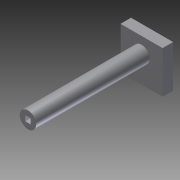
# Autodesk Inventor part: linac arm2
Saved by Autodesk Inventor 2011 (Build 150239000, 239)
## iProperties
Created: 2011-10-08
Part Number: linac arm2
Document SubType Name: Modeling
Designer: Matthew
Density: 1 g/cm^3
Author: Matthew
Autodesk Inventor part; units mm, degrees
ref_plane "YZ Plane" through (0, 0, 0) normal (1, 0, 0) x (0, 1, 0)
ref_plane "XZ Plane" through (0, 0, 0) normal (0, 1, 0) x (-1, 0, 0)
ref_plane "XY Plane" through (0, 0, 0) normal (0, 0, 1) x (1, 0, 0)
sketch "Sketch1" plane through (0, 0, 0) normal (0, 0, 1) x (1, 0, 0)
  circle A0 centre (0, 0) radius 9.906
  dimension "d0" = 19.812
  constraints: 1 centre point, 1 coincident
  measures "d0" diameter of A0
extrude "Extrusion1" add sketch "Sketch1" along normal blind 149.86
sketch "Sketch2" plane through (0, 0, 149.86) normal (0, 0, 1) x (1, 0, 0)
  circle A0 centre (0, 0) radius 9.906 projected
  circle A1 centre (0, 0) radius 3.175
  line L0 (-3.175, 0) -> (0, 0)
  line L1 (0, 0) -> (0, 3.175)
  line L2 (0, 3.175) -> (-3.175, 3.175)
  line L3 (-3.175, 3.175) -> (-3.175, 0)
  line L4 (-3.175, 3.175) -> (3.175, 3.175)
  line L5 (3.175, 3.175) -> (3.175, -3.175)
  line L6 (3.175, -3.175) -> (-3.175, -3.175)
  line L7 (-3.175, -3.175) -> (-3.175, 3.175)
  dimension "d3" = 6.35
  constraints: 16 end point, 4 parallel, 2 horizontal, 2 perpendicular, 2 point on circle, 1 centre point, 1 coincident
  measures "d3" diameter of A1
extrude "Extrusion2" cut sketch "Sketch2" against normal blind 12.7 contours A1 L0 L1 | L5 L6 A1 | A1 L4 L5 | L1 L0 A1 | A1 L3 L2 | L6 L7 A1
sketch "Sketch3" plane through (0, 0, 0) normal (0, 0, -1) x (-1, 0, 0)
  circle A0 centre (0, 0) radius 9.906 projected
  line L0 (0, 0) -> (-25.4, 0)
  line L1 (-25.4, 0) -> (-25.4, 25.4)
  line L2 (-25.4, 25.4) -> (0, 25.4)
  line L3 (0, 25.4) -> (0, 0)
  line L4 (-25.4, 25.4) -> (25.4, 25.4)
  line L5 (25.4, 25.4) -> (25.4, -25.4)
  line L6 (25.4, -25.4) -> (-25.4, -25.4)
  line L7 (-25.4, -25.4) -> (-25.4, 25.4)
  dimension "d6" = 25.4
  dimension "d7" = 25.4
  dimension "d8" = 50.8
  dimension "d9" = 50.8
  constraints: 16 end point, 4 parallel, 2 horizontal, 2 perpendicular
  measures "d6" distance of L1.end L2.end
  measures "d7" distance of L0.end L1.end
  measures "d8" distance of L5.end L6.end
  measures "d9" distance of L4.end L5.end
extrude "Extrusion3" add sketch "Sketch3" against normal blind 12.7 contours A0 L3 L4 L5 L6 L7 L0 | A0 L0 L1 L2 L3
sketch "Sketch4" plane through (-25.4, 25.4, 0) normal (0, 1, 0) x (1, 0, 0)
  line L0 (0, -12.7) -> (50.8, -12.7) projected
  line L1 (50.8, 0) -> (50.8, -12.7) projected
  line L2 (0, 0) -> (50.8, 0) projected
  line L3 (0, 0) -> (0, -12.7) projected
  point P0 (25.4, 0)
extrude "Extrusion4" cut sketch "Sketch4" against normal blind 6.35
sketch "Sketch5" plane through (0, 0, 0) normal (0, 0, -1) x (-1, 0, 0)
  line L0 (25.4, 19.05) -> (-25.4, 19.05) projected
  line L1 (-25.4, 19.05) -> (-25.4, -25.4) projected
  line L2 (-25.4, -25.4) -> (25.4, -25.4) projected
  line L3 (25.4, -25.4) -> (25.4, 19.05) projected
  line L4 (-25.4, 19.05) -> (25.4, 19.05)
  line L5 (25.4, 19.05) -> (25.4, -31.75)
  line L6 (25.4, -31.75) -> (-25.4, -31.75)
  line L7 (-25.4, -31.75) -> (-25.4, 19.05)
  point P0 (0, 0)
  dimension "d14" = 50.8
  constraints: 8 end point, 2 parallel, 1 horizontal, 1 perpendicular
  measures "d14" distance of L4.end L5.end
extrude "Extrusion5" add sketch "Sketch5" against normal blind 12.7 contours L5 L6 L7 L2
body "Solid1"
